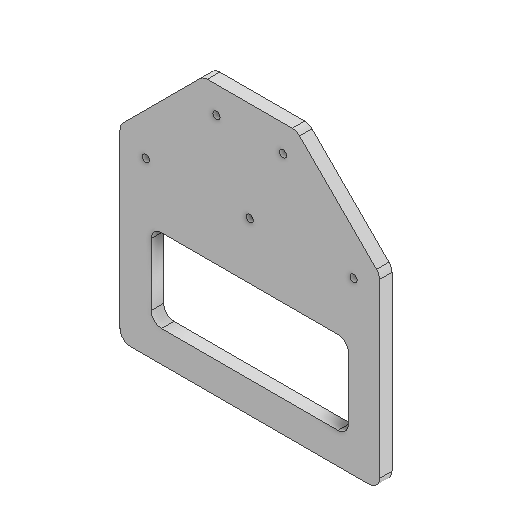
# Autodesk Inventor part: 3DP_PLA_Handle
Saved by Autodesk Inventor 2026.1 (Build 301233000, 233)
## iProperties
Created: 2025-10-19
Part Number: 3DP_PLA_Handle
Material: Generic
Document SubType Name: Modeling
Designer: User
Density: 1 g/cm^3
Appearance: Default
Author: User
Autodesk Inventor part; units mm, degrees
ref_plane "YZ Plane" through (0, 0, 0) normal (1, 0, 0) x (0, 1, 0)
ref_plane "XZ Plane" through (0, 0, 0) normal (0, 1, 0) x (-1, 0, 0)
ref_plane "XY Plane" through (0, 0, 0) normal (0, 0, 1) x (1, 0, 0)
sketch "Sketch1" plane through (0, 0, 0) normal (0, 0, 1) x (1, 0, 0)
  line L0 (-62.5, 65.8108) -> (62.5, 65.8108)
  line L1 (62.5, 65.8108) -> (62.5, -64.1892)
  line L2 (62.5, -64.1892) -> (-62.5, -64.1892)
  line L3 (-62.5, -64.1892) -> (-62.5, 65.8108)
  line L4 (-47.5, -9.1892) -> (47.5, -9.1892)
  line L5 (47.5, -9.1892) -> (47.5, -49.1892)
  line L6 (47.5, -49.1892) -> (-47.5, -49.1892)
  line L7 (-47.5, -49.1892) -> (-47.5, -9.1892)
  line L8 (-62.5, 5.8108) -> (62.5, 5.8108)
  point P0 (0, 0)
  point P1 (-50, 18)
  point P2 (50, 18)
  point P3 (0, 18)
  dimension "d0" = 125
  dimension "d1" = 62.5
  dimension "d2" = 60
  dimension "d3" = 15
  dimension "d4" = 40
  dimension "d5" = 15
  dimension "d6" = 15
  dimension "d7" = 15
  dimension "d8" = 100
  dimension "d9" = 12.5
  dimension "d24" = 50
  constraints: 18 end point, 4 parallel, 3 horizontal, 2 perpendicular, 2 point on line
  measures "d0" distance of L0.start L0.end
  measures "d1" distance from line of L3 point (0, 0)
  measures "d2" distance between parallel lines of L0 L8
  measures "d3" distance between parallel lines of L8 L4
  measures "d4" distance between parallel lines of L6 L4
  measures "d5" distance between parallel lines of L3 L7
  measures "d6" distance between parallel lines of L1 L5
  measures "d7" distance between parallel lines of L2 L6
  measures "d8" distance of point (50, 18) point (-50, 18)
  measures "d9" distance from line of L3 point (-50, 18)
  measures "d24" distance of point (0, 18) point (50, 18)
extrude "Extrusion1" add sketch "Sketch1" along normal blind 6
hole "Hole1" at (-50, 18, 0) at (50, 18, 0) at (0, 18, 0) direction (0, 0, 1) diameter 3.5 end through all
chamfer "Chamfer1" distance 40 angle 45 2 edges at (-62.5, 65.8108, 3) (62.5, 65.8108, 3)
fillet "Fillet1" radius 5 6 edges at (47.5, -9.1892, 3) (47.5, -49.1892, 3) (62.5, -64.1892, 3) (-62.5, -64.1892, 3) (-47.5, -49.1892, 3) (-47.5, -9.1892, 3)
fillet "Fillet2" radius 5 4 edges at (-62.5, 25.8108, 3) (-22.5, 65.8108, 3) (22.5, 65.8108, 3) (62.5, 25.8108, 3)
sketch "Sketch2" plane through (0, 0, 6) normal (0, 0, 1) x (1, 0, 0)
  circle A0 centre (0, 18) radius 1.75 projected
  circle A1 centre (50, 18) radius 1.75 projected
  circle A2 centre (-50, 18) radius 1.75 projected
  arc A3 (62.5, 23.7397) -> (61.0355, 27.2753) centre (57.5, 23.7397) ccw projected
  line L0 (23.9645, 64.3463) -> (61.0355, 27.2753) projected
  arc A4 (23.9645, 64.3463) -> (20.4289, 65.8108) centre (20.4289, 60.8108) ccw projected
  line L1 (20.4289, 65.8108) -> (-20.4289, 65.8108) projected
  arc A5 (-20.4289, 65.8108) -> (-23.9645, 64.3463) centre (-20.4289, 60.8108) ccw projected
  line L2 (-61.0355, 27.2753) -> (-23.9645, 64.3463) projected
  arc A6 (-61.0355, 27.2753) -> (-62.5, 23.7397) centre (-57.5, 23.7397) ccw projected
  line L3 (-62.5, 23.7397) -> (-62.5, -59.1892) projected
  arc A7 (-62.5, -59.1892) -> (-57.5, -64.1892) centre (-57.5, -59.1892) ccw projected
  line L4 (-57.5, -64.1892) -> (57.5, -64.1892) projected
  arc A8 (57.5, -64.1892) -> (62.5, -59.1892) centre (57.5, -59.1892) ccw projected
  line L5 (62.5, -59.1892) -> (62.5, 23.7397) projected
  line L6 (-42.5, -9.1892) -> (42.5, -9.1892) projected
  arc A9 (47.5, -14.1892) -> (42.5, -9.1892) centre (42.5, -14.1892) ccw projected
  line L7 (47.5, -14.1892) -> (47.5, -44.1892) projected
  arc A10 (42.5, -49.1892) -> (47.5, -44.1892) centre (42.5, -44.1892) ccw projected
  line L8 (42.5, -49.1892) -> (-42.5, -49.1892) projected
  arc A11 (-47.5, -44.1892) -> (-42.5, -49.1892) centre (-42.5, -44.1892) ccw projected
  line L9 (-47.5, -44.1892) -> (-47.5, -14.1892) projected
  arc A12 (-42.5, -9.1892) -> (-47.5, -14.1892) centre (-42.5, -14.1892) ccw projected
  point P0 (0, 0)
  point P1 (16, 53)
  point P2 (-16, 53)
  dimension "d25" = 16
  dimension "d26" = 16
  dimension "d27" = 35
  constraints: 1 horizontal alignment
  measures "d25" horizontal distance of point (0, 0) point (16, 53)
  measures "d26" horizontal distance of point (0, 0) point (-16, 53)
  measures "d27" vertical distance of A0.centre point (-16, 53)
hole "Hole2" at (16, 53, 6) at (-16, 53, 6) direction (0, 0, -1) diameter 3.5 end through all
equation "\"d1\" = 0.5 * d0"
equation "\"d5\" = d3"
equation "\"d6\" = d3"
equation "\"d7\" = d5"
equation "\"d9\" = -0.5 * d8 + 0.5 * d0"
equation "\"d24\" = 0.5 * d8"
equation "\"d26\" = d25"
body "Solid1"
